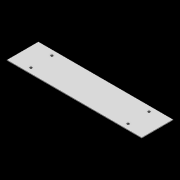
# Autodesk Inventor part: shortsidepanel
Saved by Autodesk Inventor 2022 (Build 260153000, 153)
## iProperties
Created: 2021-10-03
Part Number: shortsidepanel
Material: Generic
Document SubType Name: Modeling
Designer: timmy
Density: 1 g/cm^3
Appearance: Default
Author: timmy
Autodesk Inventor part; units mm, degrees
ref_plane "YZ Plane" through (0, 0, 0) normal (1, 0, 0) x (0, 1, 0)
ref_plane "XZ Plane" through (0, 0, 0) normal (0, 1, 0) x (-1, 0, 0)
ref_plane "XY Plane" through (0, 0, 0) normal (0, 0, 1) x (1, 0, 0)
sketch "Sketch1" plane through (0, 0, 0) normal (0, 1, 0) x (-1, 0, 0)
  line L0 (0, 0) -> (383.54, 0)
  line L1 (383.54, 0) -> (383.54, -89.5604)
  line L2 (383.54, -89.5604) -> (0, -89.5604)
  line L3 (0, -89.5604) -> (0, 0)
  dimension "d0" = 383.54
  dimension "d1" = 89.5604
  constraints: 8 end point, 2 parallel, 1 horizontal, 1 perpendicular
  measures "d0" distance of L1.end L2.end
  measures "d1" distance of L0.end L1.end
extrude "Extrusion1" add sketch "Sketch1" along normal blind 1.5875
sketch "Sketch2" plane through (0, 1.5875, 0) normal (0, 1, 0) x (1, 0, 0)
  line L0 (0, 0) -> (0, 89.5604) projected
  line L1 (-383.54, 0) -> (0, 0) projected
  circle A0 centre (-53.4416, 14.986) radius 3.175
  circle A1 centre (-53.4416, 74.5744) radius 3.175
  line L2 (-191.77, 0) -> (-191.77, 32.4011)
  circle A2 centre (-330.0984, 14.986) radius 3.175
  circle A3 centre (-330.0984, 74.5744) radius 3.175
  dimension "d6" = 6.35
  constraints: 4 centre point, 2 end point, 2 symmetric about line, 1 midpoint, 1 vertical, 2 other
  measures "d6" diameter of A0
extrude "Extrusion2" cut sketch "Sketch2" against normal blind 6.35
equation "\"d7\" = d6"
body "Solid1"
